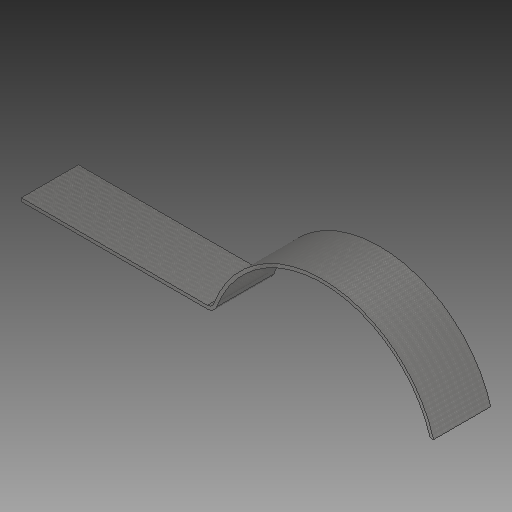
# Autodesk Inventor part: carril1
Saved by Autodesk Inventor 2019 (Build 230136000, 136)
## iProperties
Created: 2019-02-26
Part Number: carril1
Material: Generic
Document SubType Name: Modeling
Designer: felix
Density: 1 g/cm^3
Appearance: Default
Mass: 2580.65 g
Surface Area: 5491.99 cm^2
Volume: 2580.65 cm^3
Author: felix
Autodesk Inventor part; units mm, degrees
ref_plane "YZ Plane" through (0, 0, 0) normal (1, 0, 0) x (0, 1, 0)
ref_plane "XZ Plane" through (0, 0, 0) normal (0, 1, 0) x (-1, 0, 0)
ref_plane "XY Plane" through (0, 0, 0) normal (0, 0, 1) x (1, 0, 0)
sketch "Sketch1" plane through (0, 0, 0) normal (0, 0, 1) x (1, 0, 0)
  arc A0 (330.1893, 100) -> (-323.606, 119.6) centre (0, 0) ccw
  line L0 (-351.7456, 100) -> (-921.7456, 100)
  arc A1 (-351.7456, 100) -> (-323.606, 119.6) centre (-351.7456, 130) ccw
  arc A2 (340.6244, 100) -> (-332.9859, 123.0667) centre (0, 0) ccw
  line L1 (-921.7456, 100) -> (-921.7456, 110)
  line L2 (-921.7456, 110) -> (-351.7456, 110)
  arc A3 (-351.7456, 110) -> (-332.9859, 123.0667) centre (-351.7456, 130) ccw
  line L3 (0, 0) -> (0, 130)
  line L4 (330.1893, 100) -> (340.6244, 100)
  point P0 (330.3407, 130)
  dimension "d25" = 130
  dimension "d26" = 20
  dimension "d27" = 30
  dimension "d28" = 570
  dimension "d29" = 345
  dimension "d30" = 100
  constraints: 10 end point, 9 point on circle, 4 centre point, 4 tangent, 3 horizontal alignment, 2 coincident, 2 concentric, 2 vertical, 1 horizontal, 1 perpendicular
  measures "d25" distance of L3.start L3.end
  measures "d26" radius of A3
  measures "d27" radius of A1
  measures "d28" distance of L0.start L0.end
  measures "d29" radius of A0
  measures "d30" distance from line of point (0, 0) L0
extrude "Extrusion1" add sketch "Sketch1" along normal blind 175
body "Solid1"
